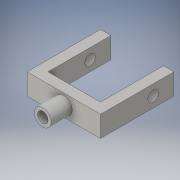
# Autodesk Inventor part: BaseFork
Saved by Autodesk Inventor 2016 (Build 200138000, 138)
## iProperties
Created: 2017-04-12
Part Number: BaseFork
Material: Generic
Document SubType Name: Modeling
Designer: Evan Phil George
Density: 1 g/cm^3
Appearance: Default
Author: Evan Phil George
Autodesk Inventor part; units mm, degrees
ref_plane "YZ Plane" through (0, 0, 0) normal (1, 0, 0) x (0, 1, 0)
ref_plane "XZ Plane" through (0, 0, 0) normal (0, 1, 0) x (-1, 0, 0)
ref_plane "XY Plane" through (0, 0, 0) normal (0, 0, 1) x (1, 0, 0)
sketch "Sketch1" plane through (0, 0, 0) normal (0, 1, 0) x (-1, 0, 0)
  line L0 (0, 0) -> (-12.5, 0)
  line L1 (0, 0) -> (12.5, 0)
  line L2 (12.5, 0) -> (12.5, -30)
  line L3 (-12.5, 0) -> (-12.5, -30)
  line L4 (12.5, -30) -> (17.5, -30)
  line L5 (17.5, -30) -> (17.5, 5)
  line L6 (-12.5, -30) -> (-17.5, -30)
  line L7 (-17.5, -30) -> (-17.5, 5)
  line L8 (-17.5, 5) -> (17.5, 5)
  dimension "d0" = 12.5
  dimension "d1" = 12.5
  dimension "d2" = 30
  dimension "d3" = 30
  dimension "d4" = 5
  dimension "d5" = 35
  dimension "d6" = 5
  dimension "d7" = 35
  constraints: 18 end point, 4 horizontal, 2 perpendicular, 2 vertical
  measures "d0" distance of L0.start L0.end
  measures "d1" distance of L0.start L1.end
  measures "d2" distance of L1.end L2.end
  measures "d3" distance of L0.end L3.end
  measures "d4" distance of L2.end L4.end
  measures "d5" distance of L4.end L5.end
  measures "d6" distance of L3.end L6.end
  measures "d7" distance of L6.end L7.end
extrude "Extrusion1" add sketch "Sketch1" along normal blind 10
sketch "Sketch2" plane through (17.5, 0, 5) normal (1, 0, 0) x (0, 0, -1)
  line L0 (35, 0) -> (35, 10) projected
  line L1 (35, 5) -> (25, 5)
  circle A0 centre (25, 5) radius 2.5
  point P0 (5, 0)
  dimension "d10" = 10
  dimension "d11" = 5
  constraints: 2 end point, 1 centre point, 1 coincident, 1 horizontal, 1 midpoint
  measures "d10" distance of L1.start L1.end
  measures "d11" diameter of A0
extrude "Extrusion2" cut sketch "Sketch2" against normal blind 35
sketch "Sketch3" plane through (-17.5, 0, 5) normal (0, 0, 1) x (1, 0, 0)
  line L0 (5, 10) -> (0, 10) projected
  line L1 (30, 0) -> (35, 0) projected
  line L2 (0, 10) -> (35, 0)
  circle A0 centre (17.5, 5) radius 4
  circle A1 centre (17.5, 5) radius 2.5
  point P0 (17.5, 0)
  dimension "d14" = 8
  dimension "d15" = 5
  constraints: 2 centre point, 2 end point, 1 coincident, 1 midpoint
  measures "d14" diameter of A0
  measures "d15" diameter of A1
extrude "Extrusion3" add sketch "Sketch3" along normal blind 10 contours A0 L2 A1 | L2 A1 A0
body "Solid1"
